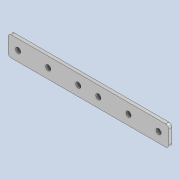
# Autodesk Inventor part: X Axis Drag Chain 2020 Connecting Bracket
Saved by Autodesk Inventor 2022 (Build 260153000, 153)
## iProperties
Created: 2021-10-30
Part Number: X Axis Drag Chain 2020 Connecting Bracket
Material: Generic
Document SubType Name: Modeling
Designer: Coy
Density: 1 g/cm^3
Appearance: Machined - Aluminum
Author: Coy
Autodesk Inventor part; units mm, degrees
ref_plane "YZ Plane" through (0, 0, 0) normal (1, 0, 0) x (0, 1, 0)
ref_plane "XZ Plane" through (0, 0, 0) normal (0, 1, 0) x (-1, 0, 0)
ref_plane "XY Plane" through (0, 0, 0) normal (0, 0, 1) x (1, 0, 0)
sketch "Sketch1" plane through (0, 0, 0) normal (0, 0, 1) x (1, 0, 0)
  line L0 (0, 0) -> (-160, 0)
  line L1 (-160, 0) -> (-160, 20)
  line L2 (-160, 20) -> (0, 20)
  line L3 (0, 20) -> (0, 0)
  line L4 (-160, 10) -> (0, 10) construction
  line L5 (-80, 20) -> (-80, 0) construction
  circle A0 centre (-150, 10) radius 2.6
  circle A1 centre (-120, 10) radius 2.6
  circle A2 centre (-90, 10) radius 2.6
  circle A3 centre (-70, 10) radius 2.6
  circle A4 centre (-40, 10) radius 2.6
  circle A5 centre (-10, 10) radius 2.6
  dimension "d0" = 160
  dimension "d1" = 20
  dimension "d2" = 5.2
  dimension "d4" = 5.2
  dimension "d5" = 5.2
  dimension "d6" = 5.2
  dimension "d7" = 5.2
  dimension "d8" = 10
  dimension "d11" = 10
  dimension "d12" = 30
  dimension "d13" = 10
  dimension "d14" = 10
  dimension "d15" = 30
  dimension "d16" = 5.2
  constraints: 12 end point, 6 centre point, 6 point on line, 4 midpoint, 2 parallel, 1 horizontal, 1 perpendicular
  measures "d0" distance of L1.end L2.end
  measures "d1" distance of L0.end L1.end
  measures "d2" diameter of A0
  measures "d4" diameter of A2
  measures "d5" diameter of A3
  measures "d6" diameter of A4
  measures "d7" diameter of A5
  measures "d8" distance of L4.start A0.centre
  measures "d11" distance from line of L5 A2.centre
  measures "d12" distance of A0.centre A1.centre
  measures "d13" distance from line of L5 A3.centre
  measures "d14" distance from line of L3 A5.centre
  measures "d15" distance of A3.centre A4.centre
  measures "d16" diameter of A1
extrude "Extrusion1" add sketch "Sketch1" along normal blind 3.175
fillet "Fillet1" radius 3.175 4 edges at (-160, 20, 1.5875) (-160, 0, 1.5875) (0, 20, 1.5875) (0, 0, 1.5875)
equation "\"d4\" = d2"
equation "\"d5\" = d2"
equation "\"d6\" = d2"
equation "\"d7\" = d2"
equation "\"d16\" = d2"
body "Solid1"
